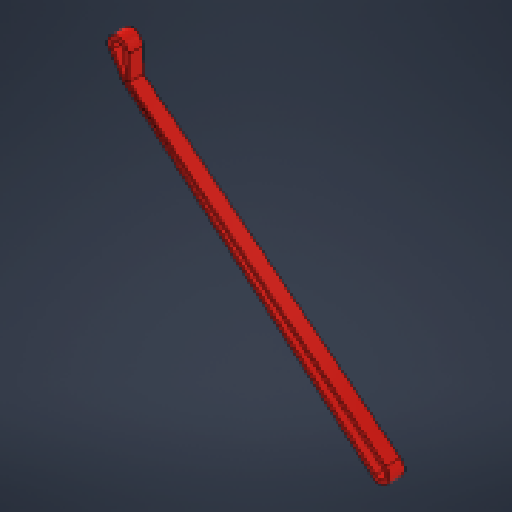
# Autodesk Inventor part: Angle Changer left band
Saved by Autodesk Inventor 2023.2 (Build 272271030, 271C)
## iProperties
Created: 2023-04-07
Part Number: Angle Changer left band
Material: Generic
Document SubType Name: Modeling
Designer: Main Account
Density: 1 g/cm^3
Appearance: Default
Author: Main Account
Autodesk Inventor part; units mm, degrees
ref_plane "YZ Plane" through (0, 0, 0) normal (1, 0, 0) x (0, 1, 0)
ref_plane "XZ Plane" through (0, 0, 0) normal (0, 1, 0) x (-1, 0, 0)
ref_plane "XY Plane" through (0, 0, 0) normal (0, 0, 1) x (1, 0, 0)
sketch "Sketch1" plane through (0, 0, 0) normal (0, 0, 1) x (1, 0, 0)
  circle A0 centre (5.9832, 5.1816) radius 2.1844 construction
  circle A1 centre (-83.8669, 86.384) radius 2.1844 construction
  line L0 (-80.2229, 78.1763) -> (-80.2229, 78.1763) construction
  line L1 (-80.2229, 78.1763) -> (-80.2229, 78.1763) construction
  line L2 (-80.2229, 78.1763) -> (-80.2229, 78.1763) construction
  line L3 (-80.2229, 78.1763) -> (-80.2229, 78.1763) construction
  line L4 (-80.2229, 78.1763) -> (-78.7415, 77.6058) construction
  line L5 (-80.2229, 78.1763) -> (-80.2229, 78.1763) construction
  arc A2 (-81.7908, 86.5502) -> (-85.6548, 85.3156) centre (-83.8669, 86.384) ccw
  arc A3 (4.6215, 3.6057) -> (7.2862, 6.8066) centre (5.9832, 5.1816) ccw
  line L6 (-81.0793, 77.6598) -> (-80.2229, 78.1763) construction
  arc A4 (3.6301, 2.4799) -> (8.2106, 7.988) centre (5.9832, 5.1816) ccw
  arc A5 (-80.2842, 86.4107) -> (-86.8371, 84.3803) centre (-83.8669, 86.384) ccw
  line L7 (-80.2229, 78.1763) -> (-80.2842, 86.4107)
  line L8 (8.2106, 7.988) -> (-80.2229, 78.1763)
  line L9 (-81.7908, 86.5502) -> (-81.0793, 77.6598)
  line L10 (-81.0793, 77.6598) -> (7.2862, 6.8066)
  line L11 (-85.6548, 85.3156) -> (-81.0798, 77.6595)
  line L12 (-81.0798, 77.6595) -> (4.6215, 3.6057)
  line L13 (3.6301, 2.4799) -> (-81.7584, 76.852)
  line L14 (-81.7584, 76.852) -> (-86.8371, 84.3803)
  point P0 (-81.5582, 83.6442)
  point P1 (-84.1592, 82.8131)
  point P2 (-87.4459, 86.5502)
extrude "Extrusion1" add sketch "Sketch1" along normal blind 5
body "Solid1"
